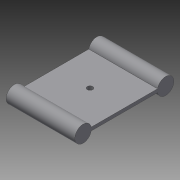
# Autodesk Inventor part: EE_Base-Rod-Rev1
Saved by Autodesk Inventor 2015 (Build 190159000, 159)
## iProperties
Created: 2016-12-22
Part Number: EE_Base-Rod-Rev1
Material: Generic
Document SubType Name: Modeling
Designer: Guy
Density: 1 g/cm^3
Appearance: Default
Author: Guy
Autodesk Inventor part; units mm, degrees
ref_plane "YZ Plane" through (0, 0, 0) normal (1, 0, 0) x (0, 1, 0)
ref_plane "XZ Plane" through (0, 0, 0) normal (0, 1, 0) x (-1, 0, 0)
ref_plane "XY Plane" through (0, 0, 0) normal (0, 0, 1) x (1, 0, 0)
sketch "Sketch1" plane through (0, 0, 0) normal (0, 0, 1) x (1, 0, 0)
  point P0 (0, 0)
sketch "Sketch2" plane through (0, 0, 0) normal (1, 0, 0) x (0, 1, 0)
  circle A0 centre (0, 0) radius 15
  circle A1 centre (0, -150) radius 15
  dimension "d0" = 30
  dimension "d1" = 30
  dimension "d2" = 150
  dimension "d3" = 0
  constraints: 2 centre point, 1 coincident
  measures "d0" diameter of A0
  measures "d1" diameter of A1
  measures "d2" distance of point (0, 0) A1.centre
  measures "d3" horizontal distance of point (0, 0) A1.centre
extrude "Extrusion1" add sketch "Sketch2" along normal blind 125
sketch "Sketch3" plane through (0, 0, 0) normal (0, 0, 1) x (1, 0, 0)
  line L0 (125, -15) -> (125, 15) projected
  line L1 (0, 15) -> (0, -15) projected
  line L2 (0, 15) -> (125, 15) projected
  line L3 (0, -15) -> (125, -15) projected
  line L4 (125, 3) -> (0, 3)
  line L5 (0, 3) -> (0, -3)
  line L6 (0, -3) -> (125, -3)
  line L7 (125, -3) -> (125, 3)
  point P0 (0, 0)
  dimension "d10" = 3
  dimension "d11" = 3
  constraints: 8 end point, 2 parallel, 2 point on line, 1 horizontal, 1 perpendicular
  measures "d10" distance of point (0, 0) L4.end
  measures "d11" distance from line of point (0, 0) L6
extrude "Extrusion2" add sketch "Sketch3" against normal blind 150 contours L6 L1 L4 L0
sketch "Sketch4" plane through (0, -3, -14.6969) normal (0, -1, 0) x (1, 0, 0)
  point P0 (0, 14.6969)
sketch "Sketch5" plane through (0, 0, 0) normal (0, 1, 0) x (-1, 0, 0)
  line L0 (-125, -14.6969) -> (0, -14.6969) projected
  line L1 (-125, -14.6969) -> (-125, -135.3031) projected
  line L2 (0, -135.3031) -> (-125, -135.3031) projected
  line L3 (0, -14.6969) -> (0, -135.3031) projected
  line L4 (0, -14.6969) -> (-125, -14.6969) projected
  line L5 (-125, -14.6969) -> (-125, -14.6969) projected
  line L6 (-125, -14.6969) -> (0, -14.6969) projected
  line L7 (0, -14.6969) -> (0, -14.6969) projected
  line L8 (0, 15) -> (-125, 15) projected
  line L9 (0, -165) -> (-125, -165) projected
  circle A0 centre (-62.5, -75) radius 5
  point P0 (0, 0)
  dimension "d18" = 10
  dimension "d19" = 90
  dimension "d20" = 62.5
  constraints: 1 centre point
  measures "d18" diameter of A0
  measures "d19" distance from line of A0.centre L8
  measures "d20" distance from line of L1 A0.centre
extrude "Extrusion3" cut sketch "Sketch5" along normal mid plane 6 contours A0
body "Solid1"
